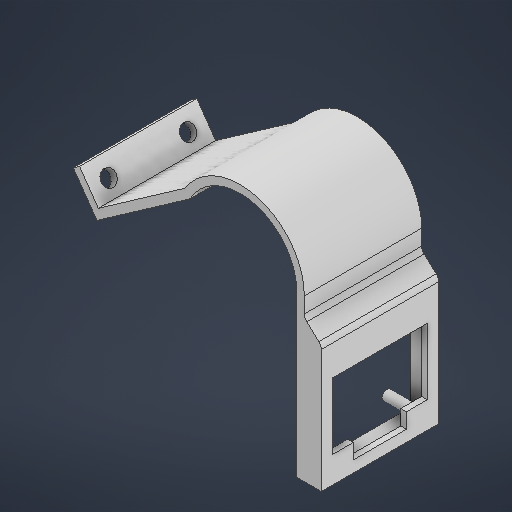
# Autodesk Inventor part: Bildschirmhalter
Saved by Autodesk Inventor 2026.2 (Build 302298000, 298)
## iProperties
Created: 2025-12-29
Part Number: Bildschirmhalter
Material: Generisch
Document SubType Name: Modeling
Designer: danie
Density: 1 g/cm^3
Appearance: Vorgabe
Author: danie
Autodesk Inventor part; units mm, degrees
ref_plane "YZ Plane" through (0, 0, 0) normal (1, 0, 0) x (0, 1, 0)
ref_plane "XZ Plane" through (0, 0, 0) normal (0, 1, 0) x (-1, 0, 0)
ref_plane "XY Plane" through (0, 0, 0) normal (0, 0, 1) x (1, 0, 0)
sketch "Skizze2" plane through (0, 0, 0) normal (1, 0, 0) x (0, 1, 0)
  line L0 (30.5, 0) -> (0, 0)
  line L1 (0, 0) -> (0, 29)
  line L2 (0, 29) -> (30.5, 29)
  line L3 (30.5, 29) -> (30.5, 0)
  line L4 (0, -5.8) -> (0, 34.8) projected
  line L5 (-26.8, 0) -> (40.05, 0) projected
  line L6 (23.5, 2) -> (7, 2)
  line L7 (7, 2) -> (7, 27)
  line L8 (7, 27) -> (23.5, 27)
  line L9 (23.5, 27) -> (23.5, 2)
  point P0 (0, 0)
  dimension "d2" = 30.5
  dimension "d3" = 29
  dimension "d4" = 2
  dimension "d5" = 2
  dimension "d6" = 7
  dimension "d7" = 7
  constraints: 16 end point, 4 parallel, 2 collinear, 2 horizontal, 2 perpendicular
  measures "d2" distance between parallel lines of L1 L3
  measures "d3" distance between parallel lines of L2 L0
  measures "d4" distance between parallel lines of L2 L8
  measures "d5" distance between parallel lines of L0 L6
  measures "d6" distance between parallel lines of L3 L9
  measures "d7" distance between parallel lines of L1 L7
extrude "Extrusion1" add sketch "Skizze2" along normal blind 1.5
sketch "Skizze4" plane through (0, 0, 0) normal (-1, 0, 0) x (0, 0, 1)
  line L0 (27, 7) -> (27, 23.5) projected
  line L1 (2, 23.5) -> (2, 7) projected
  line L2 (27, 23.5) -> (2, 23.5) projected
  line L3 (2, 7) -> (27, 7) projected
  circle A0 centre (4.25, 26.5) radius 1.25
  circle A1 centre (24.75, 26.5) radius 1.25
  circle A2 centre (4.25, 4) radius 1.25
  circle A3 centre (24.75, 4) radius 1.25
  point P0 (0, 0)
  dimension "d24" = 2.5
  dimension "d25" = 3
  dimension "d28" = 20.5
  dimension "d31" = 22.5
  dimension "d34" = 2.25
  constraints: 4 centre point, 1 horizontal, 1 vertical, 6 other
  measures "d24" diameter of A0
  measures "d25" distance from line of L2 A0.centre
  measures "d28" distance of A0.centre A1.centre
  measures "d31" distance of A0.centre A2.centre
  measures "d34" distance from line of L1 A0.centre
extrude "Extrusion2" add sketch "Skizze4" along normal blind 7 contours A0 | A1 | A2 | A3
sketch "Skizze5" plane through (0, 0, 0) normal (-1, 0, 0) x (0, 0, 1)
  line L0 (7.5, 7) -> (21.5, 7)
  line L1 (21.5, 7) -> (21.5, 2)
  line L2 (21.5, 2) -> (7.5, 2)
  line L3 (7.5, 2) -> (7.5, 7)
  line L4 (2, 7) -> (27, 7) projected
  circle A0 centre (4.25, 4) radius 1.25 projected
  circle A1 centre (24.75, 4) radius 1.25 projected
  line L5 (29, 0) -> (0, 0) projected
  dimension "d35" = 2
  dimension "d36" = 2
  dimension "d37" = 2
  constraints: 8 end point, 2 parallel, 1 collinear, 1 horizontal, 1 perpendicular
  measures "d35" distance edge to line of A0 L3
  measures "d36" distance edge to line of A1 L1
  measures "d37" distance between parallel lines of L5 L2
extrude "Extrusion3" cut sketch "Skizze5" against normal through all contours L0 L1 L2 L3
sketch "Skizze6" plane through (0, 0, 0) normal (-1, 0, 0) x (0, 0, 1)
  line L0 (2, 7) -> (7.5, 7) projected
  line L1 (7.5, 2) -> (7.5, 7) projected
  line L2 (2, 7) -> (7.5, 7)
  line L3 (7.5, 7) -> (7.5, 6)
  line L4 (7.5, 6) -> (2, 6)
  line L5 (2, 6) -> (2, 7)
  line L6 (27, 7) -> (21.5, 7)
  line L7 (21.5, 7) -> (21.5, 6)
  line L8 (21.5, 6) -> (27, 6)
  line L9 (27, 6) -> (27, 7)
  line L10 (21.5, 7) -> (21.5, 2) projected
  point P0 (0, 0)
  dimension "d40" = 1
  constraints: 16 end point, 4 parallel, 3 point on line, 2 horizontal, 2 perpendicular, 1 coincident, 1 collinear
  measures "d40" distance between parallel lines of L0 L4
extrude "Extrusion4" cut sketch "Skizze6" against normal through all
sketch "Skizze8" plane through (1.5, 0, 0) normal (1, 0, 0) x (0, 0, -1)
  line L0 (-30, 31.5) -> (1, 31.5)
  line L1 (1, 31.5) -> (1, -1)
  line L2 (1, -1) -> (-30, -1)
  line L3 (-30, -1) -> (-30, 31.5)
  line L4 (-29, 0) -> (0, 0) projected
  line L5 (0, 0) -> (0, 30.5) projected
  line L6 (0, 30.5) -> (-29, 30.5) projected
  line L7 (-29, 30.5) -> (-29, 0) projected
  line L8 (-29, 30.5) -> (0, 30.5)
  line L9 (0, 30.5) -> (0, 0)
  line L10 (0, 0) -> (-29, 0)
  line L11 (-29, 0) -> (-29, 30.5)
  dimension "d43" = 1
  dimension "d44" = 1
  dimension "d45" = 1
  dimension "d46" = 1
  constraints: 16 end point, 4 parallel, 2 horizontal, 2 perpendicular
  measures "d43" distance between parallel lines of L4 L2
  measures "d44" distance between parallel lines of L5 L1
  measures "d45" distance between parallel lines of L6 L0
  measures "d46" distance between parallel lines of L7 L3
extrude "Extrusion5" add sketch "Skizze8" against normal blind 6.5
sketch "Skizze9" plane through (1.5, -1, -1) normal (0, 0, -1) x (-1, 0, 0)
  line L0 (6.5, 32.5) -> (6.5, 0) projected
  line L1 (0, 32.5) -> (6.5, 32.5) projected
  line L2 (0, 0) -> (0, 32.5) projected
  line L3 (0, 32.5) -> (6.5, 32.5)
  line L4 (6.5, 32.5) -> (6.5, 37.5)
  line L5 (0, 31.7695) -> (0, 32.5)
  line L6 (6.5, 37.5) -> (4.5, 37.5)
  line L7 (3.8504, 36.9054) -> (0.6496, 33.9752)
  arc A0 (0.6496, 33.9752) -> (0, 32.5) centre (2, 32.5) ccw
  line L8 (4.5, 38.3806) -> (4.5, 42.5)
  line L9 (4.5, 42.5) -> (6.5, 42.5)
  line L10 (6.5, 42.5) -> (6.5, 37.5)
  arc A1 (3.8504, 36.9054) -> (4.5, 38.3806) centre (2.5, 38.3806) ccw
  point P0 (1.5, 1)
  point P1 (-0.2652, 33.1379)
  dimension "d58" = 2
  dimension "d60" = 2
  dimension "d61" = 5
  dimension "d62" = 2
  dimension "d63" = 10
  constraints: 16 end point, 4 point on circle, 4 point on line, 3 perpendicular, 3 tangent, 2 centre point, 2 horizontal, 2 vertical
  measures "d58" distance of L4.end L6.end
  measures "d60" radius of A0
  measures "d61" distance between parallel lines of L1 L6
  measures "d62" radius of A1
  measures "d63" distance between parallel lines of L1 L9
extrude "Extrusion6" add sketch "Skizze9" against normal blind 31
sketch "Skizze12" plane through (1.5, -1, -1) normal (0, 0, -1) x (-1, 0, 0)
  circle A0 centre (21.5, 42.5) radius 15
  circle A1 centre (21.5, 42.5) radius 17
  line L0 (4.5, 42.5) -> (4.5, 38.3806) projected
  line L1 (6.5, 42.5) -> (4.5, 42.5) projected
  line L2 (4.5, 42.5) -> (38.5, 42.5)
  point P0 (1.5, 1)
  point P1 (36.5, 42.5)
  dimension "d64" = 30
  constraints: 2 end point, 2 point on circle, 1 centre point, 1 collinear, 1 tangent, 4 other
extrude "Extrusion7" add sketch "Skizze12" against normal blind 31 contours A0 L1 A1 L2 picked at (5.4766, 45.0527)
sketch "Skizze13" plane through (1.5, -1, -1) normal (0, 0, -1) x (-1, 0, 0)
  line L0 (0, 0) -> (6.5, 0) projected
  line L1 (0, 0) -> (35.9872, 51.395)
  arc A0 (38.5, 42.5) -> (4.5, 42.5) centre (21.5, 42.5) ccw projected
  line L2 (0, 0) -> (0, 32.5) projected
  arc A1 (38.5, 42.5) -> (35.9872, 51.395) centre (21.5, 42.5) ccw
  arc A2 (36.5, 42.5) -> (6.5, 42.5) centre (21.5, 42.5) ccw projected
  line L3 (38.5, 42.5) -> (36.5, 42.5)
  arc A3 (36.5, 42.5) -> (34.7206, 49.5862) centre (21.5, 42.5) ccw
  point P0 (1.5, 1)
  dimension "d67" = 35
  constraints: 6 point on circle, 4 end point, 3 concentric, 2 centre point, 1 horizontal, 1 point on line
  measures "d67" angle of L1 L2
extrude "Extrusion8" cut sketch "Skizze13" against normal through all
sketch "Skizze14" plane through (1.5, -1, -1) normal (0, 0, -1) x (-1, 0, 0)
  arc A0 (34.7206, 49.5862) -> (6.5, 42.5) centre (21.5, 42.5) ccw projected
  circle A1 centre (21.5, 42.5) radius 15
  line L0 (34.7206, 49.5862) -> (59.2848, 32.3862)
  line L1 (59.2848, 32.3862) -> (60.5513, 34.195)
  arc A2 (35.9872, 51.395) -> (4.5, 42.5) centre (21.5, 42.5) ccw projected
  line L2 (60.5513, 34.195) -> (35.9872, 51.395)
  line L3 (34.7206, 49.5862) -> (35.9872, 51.395) projected
  line L4 (60.5513, 34.195) -> (65.5248, 41.2979)
  line L5 (65.5248, 41.2979) -> (63.8865, 42.445)
  line L6 (63.8865, 42.445) -> (58.913, 35.3422)
  point P0 (1.5, 1)
  dimension "d70" = 90
  dimension "d72" = 2
  dimension "d73" = 17.2
  dimension "d74" = 90
  dimension "d76" = 8.25
  constraints: 12 end point, 3 perpendicular, 1 centre point, 1 coincident, 1 concentric, 1 parallel, 1 point on line
  measures "d70" angle of L3 L0
  measures "d72" distance between parallel lines of L6 L4
  measures "d73" vertical distance of L0.end L0.start
  measures "d74" angle of L2 L4
  measures "d76" vertical distance of L1.end L5.end
extrude "Extrusion9" add sketch "Skizze14" against normal blind 31 contours L3 L2 L1 L0 | L2 L6 L5 L4
sketch "Skizze15" plane through (-62.3865, 41.445, 30) normal (0.819152, 0.5735764, 0) x (0, 0, -1)
  circle A0 centre (26, -4.671) radius 2
  circle A1 centre (5, -4.671) radius 2
  line L0 (31, 0) -> (31, -8.671) projected
  line L1 (0, -8.671) -> (0, 0) projected
  line L2 (31, -8.671) -> (0, -8.671) projected
  point P0 (30, -69.7332)
  point P1 (31, -4.3355)
  dimension "d79" = 4
  dimension "d80" = 4
  dimension "d82" = 5
  dimension "d83" = 4
  dimension "d84" = 4
  dimension "d85" = 5
  constraints: 2 centre point, 1 midpoint
  measures "d79" diameter of A0
  measures "d80" diameter of A1
  measures "d82" distance from line of L1 A1.centre
  measures "d83" distance from line of L2 A0.centre
  measures "d84" distance from line of L2 A1.centre
  measures "d85" distance from line of L0 A0.centre
extrude "Extrusion10" cut sketch "Skizze15" against normal through all
